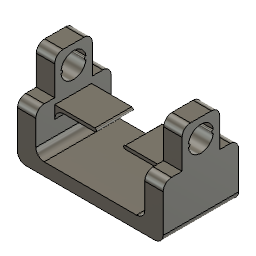
OMEGA ABOVE ALL TOOTHBRUSH HOLDERS (Autodesk Fusion 360 archive; units mm, degrees)
design "body toothbrush"
Autodesk Fusion 360 part; units mm, degrees
note: some values were not read from the file. Set by a fixed rule: which face or edge a step refers to.
sketch "Sketch1" plane through (0, 0, 0) normal (0, 1, 0) x (1, 0, 0)
sketch "Sketch2" plane through (0, 0, 0) normal (0, 1, 0) x (1, 0, 0)
  line L0 (30, 0) -> (110, 0)
  line L1 (110, 0) -> (110, -30)
  line L2 (110, -30) -> (30, -30)
  line L3 (30, -30) -> (30, 0)
  constraint horizontal L0
  constraint vertical L1
  constraint horizontal L2
  constraint vertical L3
extrude "Extrude1" add sketch "Sketch2" along normal blind 10
sketch "Sketch3" plane through (0, 10, 0) normal (0, 1, 0) x (-1, 0, 0)
  line L0 (-30, 30) -> (-110, 30)
  line L1 (-110, 30) -> (-110, 0)
  line L2 (-110, 0) -> (-30, 0)
  line L3 (-30, 0) -> (-30, 30)
  line L4 (-95, 30) -> (-110, 30)
  line L5 (-110, 30) -> (-110, 0)
  line L6 (-110, 0) -> (-95, 0)
  line L7 (-95, 0) -> (-95, 30)
  line L8 (-45, 30) -> (-30, 30)
  line L9 (-30, 30) -> (-30, 0)
  line L10 (-30, 0) -> (-45, 0)
  line L11 (-45, 0) -> (-45, 30)
  constraint horizontal L4
  constraint vertical L5
  constraint horizontal L6
  constraint vertical L7
  constraint coincident L1.end L2.start
  constraint coincident L0 L4.start
  constraint horizontal L8
  constraint vertical L9
  constraint horizontal L10
  constraint vertical L11
  constraint coincident L2.end L3.start
  constraint coincident L0 L8.start
extrude "Extrude2" add sketch "Sketch3" along normal blind 20 contours L0 L2 L3 L8 L9 L10 L11 | L0 L1 L2 L4 L5 L6 L7
sketch "Sketch4" plane through (0, 30, 0) normal (0, 1, 0) x (-1, 0, 0)
  line L0 (-95, 0) -> (-95, 30)
  line L1 (-95, 30) -> (-110, 30)
  line L2 (-110, 30) -> (-110, 0)
  line L3 (-110, 0) -> (-95, 0)
  line L4 (-45, 30) -> (-45, 0) construction
  line L5 (-45, 0) -> (-45, 15)
  line L6 (-45, 30) -> (-30, 30) construction
  line L7 (-30, 30) -> (-37.5, 15) construction
  line L8 (-45, 7.5) -> (-30, 7.5)
  line L9 (-30, 7.5) -> (-30, 22.5)
  line L10 (-30, 22.5) -> (-45, 22.5)
  line L11 (-45, 22.5) -> (-45, 7.5)
  line L12 (-45, 7.5) -> (-30, 22.5) construction
  line L13 (-30, 7.5) -> (-45, 22.5) construction
  line L14 (-95, 7.5) -> (-110, 7.5)
  line L15 (-110, 7.5) -> (-110, 22.5)
  line L16 (-110, 22.5) -> (-95, 22.5)
  line L17 (-95, 22.5) -> (-95, 7.5)
  line L18 (-95, 7.5) -> (-110, 22.5) construction
  line L19 (-110, 7.5) -> (-95, 22.5) construction
  point P0 (-37.5, 15)
  point P1 (-102.5, 15)
  constraint vertical L4
  constraint midpoint L4 L5.end
  constraint perpendicular L4 L6
  constraint horizontal L8
  constraint perpendicular L8 L9
  constraint parallel L8 L10
  constraint parallel L9 L11
  constraint coincident L12 P0
  constraint coincident L13 P0
  constraint midpoint L5 L8.start
  constraint coincident P0 L7.end
  constraint horizontal L14
  constraint perpendicular L14 L15
  constraint parallel L14 L16
  constraint parallel L15 L17
  constraint coincident L18 P1
  constraint coincident L19 P1
  constraint coincident L0 L14.start
extrude "Extrude3" add sketch "Sketch4" along normal blind 15 contours L0 L2 L14 L15 L16 L17 | L5 L8 L9 L10 L11
sketch "Sketch5" plane through (45, 0, 0) normal (1, 0, 0) x (0, 0, -1)
  line L0 (-30, 10) -> (0, 10)
  line L1 (0, 10) -> (0, 30)
  line L2 (0, 30) -> (-7.5, 30)
  line L3 (-7.5, 30) -> (-7.5, 45)
  line L4 (-7.5, 45) -> (-22.5, 45)
  line L5 (-22.5, 45) -> (-22.5, 30)
  line L6 (-22.5, 30) -> (-30, 30)
  line L7 (-30, 30) -> (-30, 10)
sketch "Sketch6" plane through (30, 0, 0) normal (-1, 0, 0) x (0, 0, 1)
  line L0 (0, 0) -> (30, 0)
  line L1 (30, 0) -> (30, 30)
  line L2 (30, 30) -> (22.5, 30)
  line L3 (22.5, 30) -> (22.5, 45)
  line L4 (22.5, 45) -> (7.5, 45)
  line L5 (7.5, 45) -> (7.5, 30)
  line L6 (7.5, 30) -> (0, 30)
  line L7 (0, 30) -> (0, 0)
  circle A0 centre (15, 37.5) radius 5
  line L8 (11, 38) -> (9.5, 38)
  line L9 (9.5, 38) -> (9.5, 37)
  line L10 (9.5, 37) -> (11, 37)
  line L11 (11, 37) -> (11, 38)
  line L12 (19, 37) -> (20.5, 37)
  line L13 (20.5, 37) -> (20.5, 38)
  line L14 (20.5, 38) -> (19, 38)
  line L15 (19, 38) -> (19, 37)
  dimension "d7" = 10
  constraint horizontal L8
  constraint vertical L9
  constraint horizontal L10
  constraint vertical L11
  constraint horizontal L12
  constraint vertical L13
  constraint horizontal L14
  constraint vertical L15
  measures "d7" diameter of A0
extrude "Extrude4" cut sketch "Sketch6" against normal blind 85 contours A0 L8 L10 L11 L12 L14 L15
sketch "Sketch7" plane through (30, 0, 0) normal (-1, 0, 0) x (0, 0, 1)
  line L0 (11, 38) -> (10.0251, 38)
  arc A0 (19.9749, 38) -> (10.0251, 38) centre (15, 37.5) ccw
  line L1 (19.9749, 38) -> (19, 38)
  line L2 (19, 38) -> (19, 37)
  line L3 (19, 37) -> (19.9749, 37)
  arc A1 (10.0251, 37) -> (19.9749, 37) centre (15, 37.5) ccw
  line L4 (10.0251, 37) -> (11, 37)
  line L5 (11, 37) -> (11, 38)
  line L6 (0, 0) -> (30, 0)
  line L7 (30, 0) -> (30, 30)
  line L8 (30, 30) -> (22.5, 30)
  line L9 (22.5, 30) -> (22.5, 45)
  line L10 (22.5, 45) -> (7.5, 45)
  line L11 (7.5, 45) -> (7.5, 30)
  line L12 (7.5, 30) -> (0, 30)
  line L13 (0, 30) -> (0, 0)
scale "Scale1" factor 1.5 about (110, 45, 7.5) bodies 1
sketch "Sketch8" plane through (-10, 0, 0) normal (-1, 0, 0) x (0, 0, 1)
  line L0 (12.75, 34.5) -> (11.2876, 34.5)
  arc A0 (26.2124, 34.5) -> (11.2876, 34.5) centre (18.75, 33.75) ccw
  line L1 (26.2124, 34.5) -> (24.75, 34.5)
  line L2 (24.75, 34.5) -> (24.75, 33)
  line L3 (24.75, 33) -> (26.2124, 33)
  arc A1 (11.2876, 33) -> (26.2124, 33) centre (18.75, 33.75) ccw
  line L4 (11.2876, 33) -> (12.75, 33)
  line L5 (12.75, 33) -> (12.75, 34.5)
  line L6 (-3.75, -22.5) -> (41.25, -22.5)
  line L7 (41.25, -22.5) -> (41.25, 22.5)
  line L8 (41.25, 22.5) -> (30, 22.5)
  line L9 (30, 22.5) -> (30, 45)
  line L10 (30, 45) -> (7.5, 45)
  line L11 (7.5, 45) -> (7.5, 22.5)
  line L12 (7.5, 22.5) -> (-3.75, 22.5)
  line L13 (-3.75, 22.5) -> (-3.75, -22.5)
fillet "Fillet1" radius 5 1 edges at (98.75, 45, 30)
fillet "Fillet2" radius 5 2 edges at (98.75, 45, 7.5) (1.25, 45, 7.5)
fillet "Fillet3" radius 5 1 edges at (1.25, 45, 30)
fillet "Fillet4" radius 5 1 edges at (98.75, 22.5, 41.25)
fillet "Fillet5" radius 5 1 edges at (98.75, 22.5, -3.75)
fillet "Fillet6" radius 5 1 edges at (1.25, 22.5, -3.75)
fillet "Fillet7" radius 5 1 edges at (1.25, 22.5, 41.25)
extrude "Extrude5" cut sketch "Sketch8" against normal blind 11.5
extrude "Extrude6" cut 1 faces at (110, -7.5, 15) along direction (-1, 0, 0) blind 11.5
extrude "Extrude7" cut 1 faces at (33.8333, -22.5, 11.25) along direction (0, 1, 0) blind 7.5
sketch "Sketch9" plane through (98.5, 0, 0) normal (1, 0, 0) x (0, 0, -1)
  line L0 (3.75, -15) -> (3.75, 17.5)
  arc A0 (3.75, 17.5) -> (-1.25, 22.5) centre (-1.25, 17.5) ccw
  line L1 (-1.25, 22.5) -> (-7.5, 22.5)
  line L2 (-7.5, 22.5) -> (-7.5, 40)
  arc A1 (-7.5, 40) -> (-12.5, 45) centre (-12.5, 40) ccw
  line L3 (-12.5, 45) -> (-25, 45)
  arc A2 (-25, 45) -> (-30, 40) centre (-25, 40) ccw
  line L4 (-30, 40) -> (-30, 22.5)
  line L5 (-30, 22.5) -> (-36.25, 22.5)
  arc A3 (-36.25, 22.5) -> (-41.25, 17.5) centre (-36.25, 17.5) ccw
  line L6 (-41.25, 17.5) -> (-41.25, -15)
  line L7 (-11.2876, 34.5) -> (-12.75, 34.5)
  line L8 (-12.75, 34.5) -> (-12.75, 33)
  line L9 (-12.75, 33) -> (-11.2876, 33)
  arc A4 (-26.2124, 33) -> (-11.2876, 33) centre (-18.75, 33.75) ccw
  line L10 (-26.2124, 33) -> (-24.75, 33)
  line L11 (-24.75, 33) -> (-24.75, 34.5)
  line L12 (-24.75, 34.5) -> (-26.2124, 34.5)
  arc A5 (-11.2876, 34.5) -> (-26.2124, 34.5) centre (-18.75, 33.75) ccw
  circle A6 centre (-18.75, 33.75) radius 7.5
  line L13 (-41.25, -15) -> (3.75, -15)
  constraint concentric A4 A6
extrude "Extrude8" cut sketch "Sketch9" against normal blind 115 contours L7 L8 L9 A6 | L7 L8 L9 A4 L10 L11 L12 A5 A6 | L10 L11 L12 A6
sketch "Sketch10" plane through (98.5, 0, 0) normal (1, 0, 0) x (0, 0, -1)
  circle A0 centre (-18.75, 33.75) radius 7.5
  line L0 (3.75, -15) -> (3.75, 17.5)
  arc A1 (3.75, 17.5) -> (-1.25, 22.5) centre (-1.25, 17.5) ccw
  line L1 (-1.25, 22.5) -> (-7.5, 22.5)
  line L2 (-7.5, 22.5) -> (-7.5, 40)
  arc A2 (-7.5, 40) -> (-12.5, 45) centre (-12.5, 40) ccw
  line L3 (-12.5, 45) -> (-25, 45)
  arc A3 (-25, 45) -> (-30, 40) centre (-25, 40) ccw
  line L4 (-30, 40) -> (-30, 22.5)
  line L5 (-30, 22.5) -> (-36.25, 22.5)
  arc A4 (-36.25, 22.5) -> (-41.25, 17.5) centre (-36.25, 17.5) ccw
  line L6 (-41.25, 17.5) -> (-41.25, -15)
  circle A5 centre (-18.75, 33.75) radius 7.5
  line L7 (-18.75, 33.75) -> (-26.25, 33.75)
  line L8 (-18.75, 33.75) -> (-11.25, 33.75)
  circle A6 centre (-26.25, 33.75) radius 1
  circle A7 centre (-11.25, 33.75) radius 1
  line L9 (-41.25, -15) -> (3.75, -15)
  dimension "d41" = 2
  dimension "d42" = 2
  constraint concentric A0 A5
  constraint coincident A0.centre A5.centre
  constraint coincident A0 L7.end
  constraint horizontal L7
  constraint coincident A0 L8.end
  constraint parallel L7 L8
  constraint coincident L7.end A6.centre
  constraint coincident L8.end A7.centre
  measures "d41" diameter of A6
  measures "d42" diameter of A7
extrude "Extrude9" add sketch "Sketch10" against normal blind 11 contours A0 A5 L8 A7 | A0 A5 L8 A7 | A0 A5 L7 A6 | A0 A5 L7 A6
extrude "Extrude10" add sketch "Sketch10" against normal blind 11 from surface at -86 contours A0 A5 L8 A7 | A0 A5 L8 A7 | A0 A5 L7 A6 | A0 A5 L7 A6
sketch "Sketch11" plane through (12.5, 0, 0) normal (1, 0, 0) x (0, 0, -1)
  arc A0 (-11.3167, 34.7478) -> (-26.1833, 34.7478) centre (-18.75, 33.75) ccw
  arc A1 (-11.3167, 34.7478) -> (-11.3167, 32.7522) centre (-11.25, 33.75) ccw
  arc A2 (-26.1833, 32.7522) -> (-11.3167, 32.7522) centre (-18.75, 33.75) ccw
  arc A3 (-26.1833, 32.7522) -> (-26.1833, 34.7478) centre (-26.25, 33.75) ccw
  line L0 (3.75, -7.5) -> (3.75, 17.5)
  arc A4 (3.75, 17.5) -> (-1.25, 22.5) centre (-1.25, 17.5) ccw
  line L1 (-1.25, 22.5) -> (-7.5, 22.5)
  line L2 (-7.5, 22.5) -> (-7.5, 40)
  arc A5 (-7.5, 40) -> (-12.5, 45) centre (-12.5, 40) ccw
  line L3 (-12.5, 45) -> (-25, 45)
  arc A6 (-25, 45) -> (-30, 40) centre (-25, 40) ccw
  line L4 (-30, 40) -> (-30, 22.5)
  line L5 (-30, 22.5) -> (-36.25, 22.5)
  arc A7 (-36.25, 22.5) -> (-41.25, 17.5) centre (-36.25, 17.5) ccw
  line L6 (-41.25, 17.5) -> (-41.25, -7.5)
  line L7 (-30, 21) -> (-8, 21)
  line L8 (-8, 21) -> (-8, 19)
  line L9 (-8, 19) -> (-30, 19)
  line L10 (-30, 19) -> (-30, 21)
  line L11 (-41.25, -7.5) -> (3.75, -7.5)
  dimension "d48" = 22
  dimension "d49" = 2
  constraint horizontal L7
  constraint vertical L8
  constraint horizontal L9
  constraint vertical L10
  measures "d48" distance of L7.start L7.end
  measures "d49" distance of L7.start L9.end
extrude "Extrude11" add sketch "Sketch11" along normal blind 30 contours L7 L8 L9 L10
extrude "Extrude12" add sketch "Sketch11" against normal blind 30 from surface at 75 contours L7 L8 L9 L10
extrude "Extrude13" add 1 faces at (87.5, 1.3333, 15.1667) along direction (-1, 0, 0) blind 5
extrude "Extrude14" add sketch "Sketch11" along normal blind 5
extrude "Extrude15" cut sketch "Sketch10" against normal blind 5
extrude "Extrude16" cut 1 faces at (1.5, -2.5, 15) along direction (1, 0, 0) blind 5
extrude "Extrude17" cut 2 faces at (98.5, 33.4969, 26.3673) (98.5, 33.4599, 11.2143) along direction (-1, 0, 0) blind 5
fillet "Fillet15" radius 5 1 edges at (93.5, -15, 18.75)
fillet "Fillet16" radius 5 1 edges at (6.5, -15, 18.75)
fillet "Fillet17" radius 5 2 edges at (82.5, -7.5, 18.75) (17.5, -7.5, 18.75)
delete_face "DeleteFace1" 1 faces at (17.5226, -2.9753, 26.25)
delete_face "DeleteFace2" 1 faces at (78.4463, -7.4096, 11.25)
extrude "Extrude18" add 1 faces at (39.1667, -7.5, 11.25) along direction (0, 1, 0) blind 5
delete_face "DeleteFace3" 1 faces at (6.5226, -10.4753, 11.25)
delete_face "DeleteFace4" 1 faces at (93.4774, -10.4753, 26.25)
extrude "Extrude19" cut 1 faces at (35.5, -15, 11.25) along direction (0, 1, 0) blind 5
fillet "Fillet22" radius 5 2 edges at (6.5, -10, 18.75) (93.5, -10, 18.75)
fillet "Fillet23" radius 5 1 edges at (17.5, -2.5, 18.75)
fillet "Fillet24" radius 5 1 edges at (82.5, -2.5, 18.75)
sketch "Sketch12" plane through (0, -10, 0) normal (0, -1, 0) x (1, 0, 0)
  line L0 (88.5, -3.75) -> (88.5, 41.25)
  line L1 (88.5, 41.25) -> (11.5, 41.25)
  line L2 (11.5, 41.25) -> (11.5, -3.75)
  line L3 (11.5, -3.75) -> (88.5, -3.75)
  circle A0 centre (20, 20) radius 2.5
  circle A1 centre (80, 20) radius 2.5
  dimension "d95" = 5
  dimension "d96" = 5
  measures "d95" diameter of A0
  measures "d96" diameter of A1
extrude "Extrude21" add 2 faces at (25.8333, 19, 15.3333) (74.1667, 19, 15.3333) along direction (0, -1, 0) blind 1
extrude "Extrude22" cut 2 faces at (65.8333, 21, 22.6667) (34.1667, 21, 22.6667) along direction (0, -1, 0) blind 1
scale "Scale2" factor 0.9 about (6.5, 22.5, 30) bodies 1
extrude "Extrude23" add 1 faces at (23.9, 18.45, 16.8) along direction (0, -1, 0) blind 1
extrude "Extrude24" add 1 faces at (59.9, 18.45, 23.4) along direction (0, -1, 0) blind 1
extrude "Extrude25" cut 2 faces at (23.9, 20.25, 23.4) (59.9, 20.25, 16.8) along direction (0, -1, 0) blind 1
fillet "Fillet33" radius 5 1 edges at (74.9, 17.45, 20.1)
fillet "Fillet34" radius 5 1 edges at (16.4, 17.45, 20.1)
extrude "Extrude26" add 2 faces at (38.9, 18.1167, 16.8) (38.9, 18.7167, 23.4) along direction (1, 0, 0) blind 1
extrude "Extrude27" add 2 faces at (52.4, 18.1167, 16.8) (52.4, 18.7167, 23.4) along direction (-1, 0, 0) blind 1
extrude "Extrude28" cut 1 faces at (39.9, 17.7833, 16.8) along direction (-1, 0, 0) blind 1
extrude "Extrude29" cut 1 faces at (51.4, 17.7833, 16.8) along direction (1, 0, 0) blind 1
extrude "Extrude30" cut 1 faces at (52.4, 17.7833, 16.8) along direction (1, 0, 0) blind 1
fillet "Fillet36" radius 0.9 4 edges at (53.4, 19.25, 20.1) (53.4, 17.45, 20.1) (38.9, 19.25, 20.1) (38.9, 17.45, 20.1)
equation "d25 = ( -23 / 2 ) * 1 mm"
equation "d27 = ( -23 / 2 ) * 1 mm"
equation "d29 = ( -15 / 2 ) * 1 mm"
